Autodesk Fusion 360 part; units mm, degrees
(part 3 of 8)
  spline S66 degree 5 poles (224.4196, 240.1258) (224.453, 240.0356) (224.5199, 239.8554) (224.6207, 239.5853) (224.756, 239.2258) (224.9266, 238.7773) (225.0987, 238.3298) (225.2723, 237.8833) (225.4474, 237.4376) (225.624, 236.993) (225.802, 236.5493) (225.9816, 236.1066) (226.1627, 235.665) (226.3454, 235.2243) (226.5295, 234.7846) (226.7152, 234.346) (226.9025, 233.9085) (227.0914, 233.472) (227.2818, 233.0365) (227.4737, 232.6022) (227.6673, 232.1689) (227.8625, 231.7368) (228.0592, 231.3057) (228.2576, 230.8758) (228.4577, 230.4471) (228.6593, 230.0195) (228.8626, 229.5931) (229.0676, 229.1679) (229.2743, 228.7439) (229.4826, 228.3212) (229.6927, 227.8997) (229.9044, 227.4794) (230.1179, 227.0605) (230.3331, 226.6428) (230.5501, 226.2264) (230.7689, 225.8114) (230.9894, 225.3978) (231.2118, 224.9856) (231.436, 224.5747) (231.6621, 224.1653) (231.89, 223.7574) (232.1198, 223.3509) (232.3515, 222.9459) (232.5851, 222.5425) (232.8207, 222.1406) (233.0583, 221.7403) (233.2979, 221.3417) (233.5396, 220.9447) (233.7833, 220.5495) (234.0292, 220.1561) (234.2772, 219.7644) (234.5273, 219.3745) (234.7796, 218.9864) (235.0342, 218.6002) (235.2911, 218.216) (235.5503, 217.8339) (235.8121, 217.454) (236.0764, 217.0763) (236.3433, 216.701) (236.6129, 216.3281) (236.8851, 215.9574) (237.1217, 215.6404) (237.3048, 215.3984) (237.4332, 215.2303) (237.5062, 215.1354) (237.5232, 215.1133) knots -1 -1 -1 -1 -1 -1 -0.98571429 -0.97142857 -0.95714286 -0.94285714 -0.92857143 -0.91428571 -0.9 -0.88571429 -0.87142857 -0.85714286 -0.84285714 -0.82857143 -0.81428571 -0.8 -0.78571429 -0.77142857 -0.75714286 -0.74285714 -0.72857143 -0.71428571 -0.7 -0.68571429 -0.67142857 -0.65714286 -0.64285714 -0.62857143 -0.61428571 -0.6 -0.58571429 -0.57142857 -0.55714286 -0.54285714 -0.52857143 -0.51428571 -0.5 -0.48571429 -0.47142857 -0.45714286 -0.44285714 -0.42857143 -0.41428571 -0.4 -0.38571429 -0.37142857 -0.35714286 -0.34285714 -0.32857143 -0.31428571 -0.3 -0.28571429 -0.27142857 -0.25714286 -0.24285714 -0.22857143 -0.21428571 -0.2 -0.18571429 -0.17142857 -0.15714286 -0.14285714 -0.13851185 -0.13851185 -0.13851185 -0.13851185 -0.13851185 -0.13851185
  spline S67 degree 3 poles (237.4436, 213.0816) (237.5821, 213.235) (237.6893, 213.4141) (237.829, 213.8032) (237.8602, 214.0095) (237.8437, 214.3779) (237.8118, 214.5377) (237.7006, 214.8421) (237.622, 214.9849) (237.5232, 215.1133) knots 0 0 0 0 0.062015 0.062015 0.12403 0.12403 0.172638 0.172638 0.221247 0.221247 0.221247 0.221247
  arc A34 (237.4436, 213.0816) -> (232.0105, 206.8863) centre (452.3696, 19.1166) ccw
  spline S68 degree 3 poles (230.0066, 206.5422) (230.1854, 206.4386) (230.3829, 206.3709) (230.7925, 206.3151) (231.0008, 206.3274) (231.3577, 206.42) (231.5074, 206.4845) (231.7821, 206.6565) (231.9054, 206.763) (232.0105, 206.8863) knots 0 0 0 0 0.062015 0.062015 0.12403 0.12403 0.172638 0.172638 0.221247 0.221247 0.221247 0.221247
  spline S69 degree 5 poles (230.0066, 206.5422) (229.9824, 206.5562) (229.8788, 206.6161) (229.6954, 206.7215) (229.4315, 206.8714) (229.0863, 207.0646) (228.6834, 207.2861) (228.2784, 207.5047) (227.8715, 207.7204) (227.4625, 207.9332) (227.0517, 208.1431) (226.639, 208.3503) (226.2246, 208.5548) (225.8085, 208.7567) (225.3908, 208.9563) (224.9716, 209.1534) (224.5509, 209.3481) (224.1287, 209.5405) (223.705, 209.7306) (223.2799, 209.9184) (222.8534, 210.1039) (222.4256, 210.2872) (221.9964, 210.4683) (221.5659, 210.6473) (221.1341, 210.8242) (220.7012, 210.9989) (220.2669, 211.1717) (219.8315, 211.3423) (219.3949, 211.511) (218.9572, 211.6777) (218.5183, 211.8423) (218.0783, 212.0051) (217.6372, 212.1659) (217.195, 212.3247) (216.7518, 212.4817) (216.3075, 212.6368) (215.8621, 212.79) (215.4158, 212.9414) (214.9685, 213.0909) (214.5202, 213.2387) (214.0709, 213.3846) (213.6206, 213.5287) (213.1695, 213.6711) (212.7173, 213.8116) (212.2643, 213.9505) (211.8104, 214.0876) (211.3556, 214.2229) (210.8999, 214.3566) (210.4433, 214.4885) (209.9859, 214.6188) (209.5276, 214.7473) (209.0685, 214.8742) (208.6086, 214.9994) (208.1479, 215.123) (207.6863, 215.2449) (207.224, 215.3651) (206.7609, 215.4838) (206.297, 215.6008) (205.8323, 215.7162) (205.3669, 215.83) (204.9008, 215.9422) (204.4339, 216.0528) (204.0598, 216.1401) (203.7789, 216.2048) (203.5914, 216.2476) (203.4977, 216.2689) knots 0.13851185 0.13851185 0.13851185 0.13851185 0.13851185 0.13851185 0.14285714 0.15714286 0.17142857 0.18571429 0.2 0.21428571 0.22857143 0.24285714 0.25714286 0.27142857 0.28571429 0.3 0.31428571 0.32857143 0.34285714 0.35714286 0.37142857 0.38571429 0.4 0.41428571 0.42857143 0.44285714 0.45714286 0.47142857 0.48571429 0.5 0.51428571 0.52857143 0.54285714 0.55714286 0.57142857 0.58571429 0.6 0.61428571 0.62857143 0.64285714 0.65714286 0.67142857 0.68571429 0.7 0.71428571 0.72857143 0.74285714 0.75714286 0.77142857 0.78571429 0.8 0.81428571 0.82857143 0.84285714 0.85714286 0.87142857 0.88571429 0.9 0.91428571 0.92857143 0.94285714 0.95714286 0.97142857 0.98571429 1 1 1 1 1 1
  arc A35 (203.4977, 216.2689) -> (197.5222, 208.4816) centre (452.3696, 19.1166) ccw
  spline S70 degree 5 poles (197.5222, 208.4816) (197.5671, 208.3965) (197.657, 208.2266) (197.7922, 207.972) (197.9733, 207.6332) (198.201, 207.2109) (198.43, 206.7896) (198.6604, 206.3695) (198.8921, 205.9506) (199.1252, 205.5328) (199.3597, 205.1162) (199.5955, 204.7007) (199.8327, 204.2864) (200.0713, 203.8734) (200.3113, 203.4615) (200.5527, 203.0509) (200.7955, 202.6415) (201.0396, 202.2334) (201.2853, 201.8266) (201.5323, 201.421) (201.7808, 201.0167) (202.0307, 200.6137) (202.282, 200.2121) (202.5348, 199.8117) (202.7891, 199.4128) (203.0448, 199.0152) (203.3021, 198.619) (203.5608, 198.2242) (203.821, 197.8308) (204.0828, 197.4388) (204.346, 197.0483) (204.6108, 196.6593) (204.8772, 196.2718) (205.1451, 195.8858) (205.4145, 195.5013) (205.6856, 195.1184) (205.9583, 194.7371) (206.2326, 194.3574) (206.5085, 193.9794) (206.786, 193.603) (207.0652, 193.2283) (207.3461, 192.8553) (207.6287, 192.484) (207.913, 192.1145) (208.199, 191.7468) (208.4868, 191.381) (208.7764, 191.017) (209.0678, 190.655) (209.3611, 190.295) (209.6562, 189.937) (209.9532, 189.581) (210.2521, 189.2271) (210.5529, 188.8753) (210.8557, 188.5257) (211.1605, 188.1783) (211.4674, 187.8333) (211.7765, 187.4907) (212.0879, 187.1508) (212.4015, 186.8136) (212.7175, 186.479) (213.0357, 186.1471) (213.3117, 185.8637) (213.5248, 185.6476) (213.6741, 185.4977) (213.7588, 185.4131) (213.7785, 185.3934) knots -1 -1 -1 -1 -1 -1 -0.98571429 -0.97142857 -0.95714286 -0.94285714 -0.92857143 -0.91428571 -0.9 -0.88571429 -0.87142857 -0.85714286 -0.84285714 -0.82857143 -0.81428571 -0.8 -0.78571429 -0.77142857 -0.75714286 -0.74285714 -0.72857143 -0.71428571 -0.7 -0.68571429 -0.67142857 -0.65714286 -0.64285714 -0.62857143 -0.61428571 -0.6 -0.58571429 -0.57142857 -0.55714286 -0.54285714 -0.52857143 -0.51428571 -0.5 -0.48571429 -0.47142857 -0.45714286 -0.44285714 -0.42857143 -0.41428571 -0.4 -0.38571429 -0.37142857 -0.35714286 -0.34285714 -0.32857143 -0.31428571 -0.3 -0.28571429 -0.27142857 -0.25714286 -0.24285714 -0.22857143 -0.21428571 -0.2 -0.18571429 -0.17142857 -0.15714286 -0.14285714 -0.13851185 -0.13851185 -0.13851185 -0.13851185 -0.13851185 -0.13851185
  spline S71 degree 3 poles (213.9648, 183.3687) (214.0821, 183.5389) (214.165, 183.7304) (214.2527, 184.1344) (214.2567, 184.3431) (214.1923, 184.7062) (214.1398, 184.8604) (213.9898, 185.1477) (213.8933, 185.279) (213.7785, 185.3934) knots 0 0 0 0 0.062015 0.062015 0.12403 0.12403 0.172638 0.172638 0.221247 0.221247 0.221247 0.221247
  arc A36 (213.9648, 183.3687) -> (209.3868, 176.5173) centre (452.3696, 19.1166) ccw
  spline S72 degree 3 poles (207.445, 175.9146) (207.6358, 175.8352) (207.8404, 175.7939) (208.2538, 175.7919) (208.4587, 175.8314) (208.8005, 175.9698) (208.9405, 176.0532) (209.1904, 176.2596) (209.2988, 176.3813) (209.3868, 176.5173) knots 0 0 0 0 0.062015 0.062015 0.12403 0.12403 0.172638 0.172638 0.221247 0.221247 0.221247 0.221247
  spline S73 degree 5 poles (207.445, 175.9146) (207.4192, 175.9253) (207.3086, 175.9712) (207.113, 176.0517) (206.8318, 176.1659) (206.4644, 176.3124) (206.036, 176.4794) (205.606, 176.6433) (205.1743, 176.804) (204.7411, 176.9616) (204.3064, 177.1161) (203.8702, 177.2676) (203.4326, 177.4163) (202.9937, 177.5622) (202.5536, 177.7055) (202.1122, 177.8462) (201.6697, 177.9843) (201.226, 178.12) (200.7812, 178.2532) (200.3352, 178.3839) (199.8881, 178.5121) (199.44, 178.638) (198.9909, 178.7616) (198.5407, 178.8828) (198.0895, 179.0018) (197.6374, 179.1186) (197.1844, 179.2331) (196.7304, 179.3455) (196.2756, 179.4558) (195.8198, 179.5638) (195.3632, 179.6698) (194.9057, 179.7737) (194.4474, 179.8756) (193.9882, 179.9754) (193.5283, 180.0731) (193.0676, 180.1689) (192.606, 180.2627) (192.1438, 180.3545) (191.6807, 180.4444) (191.217, 180.5324) (190.7525, 180.6184) (190.2873, 180.7025) (189.8214, 180.7847) (189.3548, 180.8651) (188.8875, 180.9436) (188.4196, 181.0203) (187.951, 181.0951) (187.4818, 181.1681) (187.0119, 181.2394) (186.5414, 181.3088) (186.0702, 181.3764) (185.5985, 181.4423) (185.1262, 181.5064) (184.6533, 181.5688) (184.1797, 181.6294) (183.7057, 181.6883) (183.231, 181.7454) (182.7558, 181.8009) (182.2801, 181.8547) (181.8038, 181.9068) (181.327, 181.9572) (180.8497, 182.0059) (180.4674, 182.0436) (180.1804, 182.0711) (179.989, 182.089) (179.8933, 182.098) knots 0.13851185 0.13851185 0.13851185 0.13851185 0.13851185 0.13851185 0.14285714 0.15714286 0.17142857 0.18571429 0.2 0.21428571 0.22857143 0.24285714 0.25714286 0.27142857 0.28571429 0.3 0.31428571 0.32857143 0.34285714 0.35714286 0.37142857 0.38571429 0.4 0.41428571 0.42857143 0.44285714 0.45714286 0.47142857 0.48571429 0.5 0.51428571 0.52857143 0.54285714 0.55714286 0.57142857 0.58571429 0.6 0.61428571 0.62857143 0.64285714 0.65714286 0.67142857 0.68571429 0.7 0.71428571 0.72857143 0.74285714 0.75714286 0.77142857 0.78571429 0.8 0.81428571 0.82857143 0.84285714 0.85714286 0.87142857 0.88571429 0.9 0.91428571 0.92857143 0.94285714 0.95714286 0.97142857 0.98571429 1 1 1 1 1 1
  arc A37 (179.8933, 182.098) -> (174.9854, 173.5973) centre (452.3696, 19.1166) ccw
  spline S74 degree 5 poles (174.9854, 173.5973) (175.041, 173.5188) (175.1523, 173.3621) (175.3196, 173.1273) (175.5433, 172.8151) (175.8242, 172.426) (176.1062, 172.0383) (176.3895, 171.6519) (176.6739, 171.2668) (176.9596, 170.883) (177.2464, 170.5005) (177.5344, 170.1194) (177.8237, 169.7396) (178.1142, 169.3612) (178.4058, 168.9842) (178.6988, 168.6086) (178.9929, 168.2344) (179.2883, 167.8617) (179.5849, 167.4904) (179.8827, 167.1205) (180.1819, 166.7521) (180.4822, 166.3852) (180.7838, 166.0198) (181.0867, 165.6559) (181.3909, 165.2935) (181.6964, 164.9327) (182.0031, 164.5735) (182.3112, 164.2158) (182.6205, 163.8598) (182.9312, 163.5053) (183.2431, 163.1525) (183.5565, 162.8014) (183.8711, 162.452) (184.1871, 162.1043) (184.5045, 161.7583) (184.8232, 161.414) (185.1433, 161.0716) (185.4648, 160.7309) (185.7877, 160.3921) (186.112, 160.0551) (186.4377, 159.7201) (186.7649, 159.3869) (187.0935, 159.0557) (187.4236, 158.7265) (187.7552, 158.3993) (188.0883, 158.0741) (188.4229, 157.7511) (188.759, 157.4302) (189.0968, 157.1116) (189.4361, 156.7952) (189.777, 156.481) (190.1196, 156.1691) (190.4637, 155.8596) (190.8096, 155.5525) (191.1571, 155.2478) (191.5064, 154.9458) (191.8576, 154.6466) (192.2106, 154.3502) (192.5656, 154.0568) (192.9226, 153.7663) (193.2814, 153.4788) (193.592, 153.2338) (193.8315, 153.0474) (193.999, 152.9183) (194.0941, 152.8455) (194.1162, 152.8285) knots -1 -1 -1 -1 -1 -1 -0.98571429 -0.97142857 -0.95714286 -0.94285714 -0.92857143 -0.91428571 -0.9 -0.88571429 -0.87142857 -0.85714286 -0.84285714 -0.82857143 -0.81428571 -0.8 -0.78571429 -0.77142857 -0.75714286 -0.74285714 -0.72857143 -0.71428571 -0.7 -0.68571429 -0.67142857 -0.65714286 -0.64285714 -0.62857143 -0.61428571 -0.6 -0.58571429 -0.57142857 -0.55714286 -0.54285714 -0.52857143 -0.51428571 -0.5 -0.48571429 -0.47142857 -0.45714286 -0.44285714 -0.42857143 -0.41428571 -0.4 -0.38571429 -0.37142857 -0.35714286 -0.34285714 -0.32857143 -0.31428571 -0.3 -0.28571429 -0.27142857 -0.25714286 -0.24285714 -0.22857143 -0.21428571 -0.2 -0.18571429 -0.17142857 -0.15714286 -0.14285714 -0.13851185 -0.13851185 -0.13851185 -0.13851185 -0.13851185 -0.13851185
  spline S75 degree 3 poles (194.5652, 150.8454) (194.6592, 151.0295) (194.7165, 151.2302) (194.7507, 151.6422) (194.7274, 151.8496) (194.6162, 152.2012) (194.544, 152.3472) (194.3578, 152.6125) (194.2449, 152.7301) (194.1162, 152.8285) knots 0 0 0 0 0.062015 0.062015 0.12403 0.12403 0.172638 0.172638 0.221247 0.221247 0.221247 0.221247
  arc A38 (194.5652, 150.8454) -> (190.9207, 143.4551) centre (452.3696, 19.1166) ccw
  spline S76 degree 3 poles (189.0741, 142.6041) (189.2737, 142.5503) (189.4819, 142.536) (189.892, 142.5881) (190.09, 142.6539) (190.4108, 142.8357) (190.5387, 142.9367) (190.7595, 143.174) (190.8511, 143.3088) (190.9207, 143.4551) knots 0 0 0 0 0.062015 0.062015 0.12403 0.12403 0.172638 0.172638 0.221247 0.221247 0.221247 0.221247
  spline S77 degree 5 poles (189.0741, 142.6041) (189.0471, 142.6113) (188.9315, 142.6424) (188.7271, 142.6967) (188.4334, 142.7732) (188.05, 142.8705) (187.6034, 142.9802) (187.1557, 143.0865) (186.7068, 143.1895) (186.2567, 143.2892) (185.8056, 143.3856) (185.3533, 143.4789) (184.9001, 143.5692) (184.4459, 143.6566) (183.9908, 143.7412) (183.5348, 143.8231) (183.0781, 143.9023) (182.6205, 143.9789) (182.162, 144.0528) (181.7028, 144.1242) (181.2429, 144.193) (180.7821, 144.2593) (180.3207, 144.3232) (179.8586, 144.3847) (179.3957, 144.4438) (178.9323, 144.5005) (178.4681, 144.555) (178.0034, 144.6071) (177.538, 144.6571) (177.0721, 144.7047) (176.6055, 144.7502) (176.1384, 144.7935) (175.6707, 144.8347) (175.2024, 144.8737) (174.7337, 144.9106) (174.2644, 144.9454) (173.7946, 144.9781) (173.3243, 145.0088) (172.8535, 145.0375) (172.3822, 145.0642) (171.9105, 145.0888) (171.4383, 145.1115) (170.9656, 145.1322) (170.4925, 145.151) (170.019, 145.1679) (169.545, 145.1828) (169.0707, 145.1958) (168.5959, 145.207) (168.1208, 145.2163) (167.6452, 145.2237) (167.1693, 145.2292) (166.693, 145.233) (166.2164, 145.2349) (165.7393, 145.235) (165.262, 145.2333) (164.7843, 145.2298) (164.3062, 145.2245) (163.8278, 145.2175) (163.3491, 145.2087) (162.8701, 145.1982) (162.3908, 145.1859) (161.9112, 145.1719) (161.5273, 145.1593) (161.2392, 145.1491) (161.0471, 145.142) (160.951, 145.1383) knots 0.13851185 0.13851185 0.13851185 0.13851185 0.13851185 0.13851185 0.14285714 0.15714286 0.17142857 0.18571429 0.2 0.21428571 0.22857143 0.24285714 0.25714286 0.27142857 0.28571429 0.3 0.31428571 0.32857143 0.34285714 0.35714286 0.37142857 0.38571429 0.4 0.41428571 0.42857143 0.44285714 0.45714286 0.47142857 0.48571429 0.5 0.51428571 0.52857143 0.54285714 0.55714286 0.57142857 0.58571429 0.6 0.61428571 0.62857143 0.64285714 0.65714286 0.67142857 0.68571429 0.7 0.71428571 0.72857143 0.74285714 0.75714286 0.77142857 0.78571429 0.8 0.81428571 0.82857143 0.84285714 0.85714286 0.87142857 0.88571429 0.9 0.91428571 0.92857143 0.94285714 0.95714286 0.97142857 0.98571429 1 1 1 1 1 1
  arc A39 (160.951, 145.1383) -> (157.1947, 136.0698) centre (452.3696, 19.1166) ccw
  spline S78 degree 5 poles (157.1947, 136.0698) (157.26, 135.9993) (157.3908, 135.8584) (157.5873, 135.6474) (157.8499, 135.3671) (158.1792, 135.018) (158.5094, 134.6704) (158.8407, 134.3243) (159.173, 133.9796) (159.5062, 133.6364) (159.8405, 133.2946) (160.1759, 132.9543) (160.5122, 132.6156) (160.8496, 132.2784) (161.188, 131.9427) (161.5274, 131.6085) (161.8679, 131.2759) (162.2094, 130.9449) (162.5519, 130.6155) (162.8955, 130.2876) (163.2402, 129.9614) (163.5858, 129.6369) (163.9326, 129.314) (164.2804, 128.9927) (164.6293, 128.6731) (164.9792, 128.3553) (165.3302, 128.0392) (165.6823, 127.7248) (166.0355, 127.4121) (166.3897, 127.1013) (166.7451, 126.7922) (167.1016, 126.485) (167.4591, 126.1796) (167.8178, 125.8761) (168.1776, 125.5745) (168.5385, 125.2748) (168.9006, 124.9771) (169.2638, 124.6813) (169.6282, 124.3875) (169.9937, 124.0958) (170.3604, 123.8061) (170.7282, 123.5185) (171.0973, 123.2331) (171.4675, 122.9497) (171.839, 122.6686) (172.2116, 122.3897) (172.5855, 122.1131) (172.9607, 121.8389) (173.3372, 121.567) (173.7149, 121.2976) (174.0939, 121.0306) (174.4742, 120.7661) (174.8558, 120.5042) (175.2388, 120.2448) (175.6231, 119.9881) (176.0089, 119.7343) (176.3961, 119.4835) (176.7848, 119.2357) (177.1751, 118.9911) (177.5668, 118.7497) (177.9602, 118.5115) (178.3001, 118.3092) (178.5618, 118.1556) (178.7448, 118.0495) (178.8485, 117.9897) (178.8727, 117.9758) knots -1 -1 -1 -1 -1 -1 -0.98571429 -0.97142857 -0.95714286 -0.94285714 -0.92857143 -0.91428571 -0.9 -0.88571429 -0.87142857 -0.85714286 -0.84285714 -0.82857143 -0.81428571 -0.8 -0.78571429 -0.77142857 -0.75714286 -0.74285714 -0.72857143 -0.71428571 -0.7 -0.68571429 -0.67142857 -0.65714286 -0.64285714 -0.62857143 -0.61428571 -0.6 -0.58571429 -0.57142857 -0.55714286 -0.54285714 -0.52857143 -0.51428571 -0.5 -0.48571429 -0.47142857 -0.45714286 -0.44285714 -0.42857143 -0.41428571 -0.4 -0.38571429 -0.37142857 -0.35714286 -0.34285714 -0.32857143 -0.31428571 -0.3 -0.28571429 -0.27142857 -0.25714286 -0.24285714 -0.22857143 -0.21428571 -0.2 -0.18571429 -0.17142857 -0.15714286 -0.14285714 -0.13851185 -0.13851185 -0.13851185 -0.13851185 -0.13851185 -0.13851185
  spline S79 degree 3 poles (179.5767, 116.0682) (179.6459, 116.263) (179.6764, 116.4695) (179.6566, 116.8824) (179.6065, 117.085) (179.4503, 117.419) (179.3596, 117.5544) (179.1404, 117.7931) (179.0131, 117.8949) (178.8727, 117.9758) knots 0 0 0 0 0.062015 0.062015 0.12403 0.12403 0.172638 0.172638 0.221247 0.221247 0.221247 0.221247
  arc A40 (179.5767, 116.0682) -> (176.928, 108.2654) centre (452.3696, 19.1166) ccw
  spline S80 degree 3 poles (175.2083, 107.1806) (175.4132, 107.1534) (175.6215, 107.1664) (176.0213, 107.2716) (176.209, 107.3627) (176.5033, 107.5848) (176.617, 107.7017) (176.8049, 107.9657) (176.8781, 108.1113) (176.928, 108.2654) knots 0 0 0 0 0.062015 0.062015 0.12403 0.12403 0.172638 0.172638 0.221247 0.221247 0.221247 0.221247
  spline S81 degree 5 poles (175.2083, 107.1806) (175.1806, 107.1843) (175.0619, 107.2) (174.8521, 107.2272) (174.551, 107.2648) (174.1582, 107.3112) (173.7011, 107.3616) (173.2433, 107.4086) (172.7848, 107.4521) (172.3256, 107.4922) (171.8657, 107.5289) (171.4051, 107.5624) (170.944, 107.5927) (170.4823, 107.6201) (170.02, 107.6446) (169.5573, 107.6662) (169.0941, 107.6852) (168.6304, 107.7013) (168.1662, 107.7148) (167.7017, 107.7257) (167.2366, 107.7338) (166.7712, 107.7395) (166.3054, 107.7426) (165.8392, 107.7432) (165.3726, 107.7413) (164.9057, 107.7371) (164.4384, 107.7305) (163.9708, 107.7216) (163.5029, 107.7103) (163.0347, 107.6968) (162.5662, 107.681) (162.0974, 107.6629) (161.6284, 107.6427) (161.1591, 107.6202) (160.6895, 107.5956) (160.2196, 107.5689) (159.7496, 107.54) (159.2793, 107.5091) (158.8088, 107.4761) (158.3381, 107.441) (157.8671, 107.4039) (157.396, 107.3647) (156.9247, 107.3236) (156.4532, 107.2804) (155.9815, 107.2353) (155.5097, 107.1883) (155.0377, 107.1393) (154.5656, 107.0884) (154.0933, 107.0355) (153.6208, 106.9808) (153.1482, 106.9242) (152.6755, 106.8658) (152.2027, 106.8054) (151.7297, 106.7433) (151.2567, 106.6793) (150.7835, 106.6134) (150.3102, 106.5458) (149.8369, 106.4764) (149.3634, 106.4052) (148.8899, 106.3323) (148.4163, 106.2575) (147.9426, 106.1811) (147.5636, 106.1185) (147.2793, 106.0708) (147.0898, 106.0386) (146.995, 106.0224) knots 0.13851185 0.13851185 0.13851185 0.13851185 0.13851185 0.13851185 0.14285714 0.15714286 0.17142857 0.18571429 0.2 0.21428571 0.22857143 0.24285714 0.25714286 0.27142857 0.28571429 0.3 0.31428571 0.32857143 0.34285714 0.35714286 0.37142857 0.38571429 0.4 0.41428571 0.42857143 0.44285714 0.45714286 0.47142857 0.48571429 0.5 0.51428571 0.52857143 0.54285714 0.55714286 0.57142857 0.58571429 0.6 0.61428571 0.62857143 0.64285714 0.65714286 0.67142857 0.68571429 0.7 0.71428571 0.72857143 0.74285714 0.75714286 0.77142857 0.78571429 0.8 0.81428571 0.82857143 0.84285714 0.85714286 0.87142857 0.88571429 0.9 0.91428571 0.92857143 0.94285714 0.95714286 0.97142857 0.98571429 1 1 1 1 1 1
  arc A41 (146.995, 106.0224) -> (144.4545, 96.5412) centre (452.3696, 19.1166) ccw
  spline S82 degree 5 poles (144.4545, 96.5412) (144.5285, 96.4798) (144.6766, 96.3572) (144.8989, 96.1737) (145.1958, 95.93) (145.5678, 95.6269) (145.9406, 95.3254) (146.3142, 95.0255) (146.6887, 94.7271) (147.0639, 94.4303) (147.44, 94.1351) (147.8168, 93.8415) (148.1945, 93.5496) (148.573, 93.2592) (148.9523, 92.9706) (149.3325, 92.6836) (149.7134, 92.3983) (150.0952, 92.1147) (150.4778, 91.8328) (150.8613, 91.5526) (151.2455, 91.2742) (151.6306, 90.9975) (152.0166, 90.7226) (152.4033, 90.4495) (152.7909, 90.1782) (153.1793, 89.9088) (153.5686, 89.6412) (153.9587, 89.3754) (154.3497, 89.1116) (154.7415, 88.8496) (155.1342, 88.5896) (155.5277, 88.3315) (155.922, 88.0754) (156.3173, 87.8213) (156.7134, 87.5693) (157.1103, 87.3192) (157.5081, 87.0713) (157.9068, 86.8255) (158.3064, 86.5818) (158.7069, 86.3402) (159.1083, 86.1009) (159.5105, 85.8638) (159.9137, 85.6289) (160.3177, 85.3963) (160.7227, 85.1661) (161.1286, 84.9382) (161.5354, 84.7128) (161.9431, 84.4899) (162.3518, 84.2695) (162.7615, 84.0517) (163.1721, 83.8365) (163.5837, 83.6239) (163.9963, 83.414) (164.4098, 83.2068) (164.8243, 83.0025) (165.2399, 82.8012) (165.6566, 82.6031) (166.0743, 82.4082) (166.4931, 82.2166) (166.9131, 82.0284) (167.3341, 81.8436) (167.6975, 81.6873) (167.9771, 81.5693) (168.1724, 81.4879) (168.283, 81.4422) (168.3088, 81.4315) knots -1 -1 -1 -1 -1 -1 -0.98571429 -0.97142857 -0.95714286 -0.94285714 -0.92857143 -0.91428571 -0.9 -0.88571429 -0.87142857 -0.85714286 -0.84285714 -0.82857143 -0.81428571 -0.8 -0.78571429 -0.77142857 -0.75714286 -0.74285714 -0.72857143 -0.71428571 -0.7 -0.68571429 -0.67142857 -0.65714286 -0.64285714 -0.62857143 -0.61428571 -0.6 -0.58571429 -0.57142857 -0.55714286 -0.54285714 -0.52857143 -0.51428571 -0.5 -0.48571429 -0.47142857 -0.45714286 -0.44285714 -0.42857143 -0.41428571 -0.4 -0.38571429 -0.37142857 -0.35714286 -0.34285714 -0.32857143 -0.31428571 -0.3 -0.28571429 -0.27142857 -0.25714286 -0.24285714 -0.22857143 -0.21428571 -0.2 -0.18571429 -0.17142857 -0.15714286 -0.14285714 -0.13851185 -0.13851185 -0.13851185 -0.13851185 -0.13851185 -0.13851185
  spline S83 degree 3 poles (169.2557, 79.6322) (169.2989, 79.8343) (169.3022, 80.043) (169.2287, 80.4498) (169.1526, 80.6441) (168.9541, 80.9549) (168.8465, 81.0773) (168.598, 81.2853) (168.4586, 81.3697) (168.3088, 81.4315) knots 0 0 0 0 0.062015 0.062015 0.12403 0.12403 0.172638 0.172638 0.221247 0.221247 0.221247 0.221247
  arc A42 (169.2557, 79.6322) -> (167.6482, 71.5504) centre (452.3696, 19.1166) ccw
  spline S84 degree 3 poles (166.0848, 70.2504) (166.2915, 70.2502) (166.4963, 70.2903) (166.879, 70.4467) (167.0532, 70.5615) (167.316, 70.8202) (167.4134, 70.9509) (167.5652, 71.2372) (167.6188, 71.3911) (167.6482, 71.5504) knots 0 0 0 0 0.062015 0.062015 0.12403 0.12403 0.172638 0.172638 0.221247 0.221247 0.221247 0.221247
  spline S85 degree 5 poles (166.0848, 70.2504) (166.0568, 70.2505) (165.9371, 70.2506) (165.7256, 70.2501) (165.4221, 70.248) (165.0266, 70.2428) (164.5669, 70.2331) (164.1069, 70.2199) (163.6466, 70.2032) (163.1861, 70.183) (162.7253, 70.1594) (162.2643, 70.1325) (161.8032, 70.1024) (161.3418, 70.0692) (160.8803, 70.0332) (160.4187, 69.9943) (159.957, 69.9526) (159.4952, 69.9081) (159.0333, 69.8609) (158.5712, 69.811) (158.1091, 69.7584) (157.6469, 69.7032) (157.1847, 69.6455) (156.7224, 69.5852) (156.26, 69.5225) (155.7977, 69.4574) (155.3353, 69.3899) (154.8728, 69.32) (154.4104, 69.2477) (153.948, 69.1732) (153.4856, 69.0964) (153.0231, 69.0173) (152.5607, 68.936) (152.0984, 68.8525) (151.636, 68.7668) (151.1737, 68.679) (150.7114, 68.589) (150.2492, 68.4969) (149.787, 68.4028) (149.3249, 68.3065) (148.8629, 68.2083) (148.4009, 68.108) (147.939, 68.0057) (147.4771, 67.9014) (147.0154, 67.7951) (146.5537, 67.6868) (146.0922, 67.5766) (145.6307, 67.4645) (145.1693, 67.3505) (144.7081, 67.2346) (144.2469, 67.1168) (143.7859, 66.9971) (143.325, 66.8756) (142.8642, 66.7522) (142.4035, 66.627) (141.943, 66.5) (141.4826, 66.3712) (141.0223, 66.2406) (140.5622, 66.1082) (140.1023, 65.9741) (139.6425, 65.8382) (139.1828, 65.7005) (138.8152, 65.589) (138.5396, 65.5046) (138.3559, 65.448) (138.264, 65.4196) knots 0.13851185 0.13851185 0.13851185 0.13851185 0.13851185 0.13851185 0.14285714 0.15714286 0.17142857 0.18571429 0.2 0.21428571 0.22857143 0.24285714 0.25714286 0.27142857 0.28571429 0.3 0.31428571 0.32857143 0.34285714 0.35714286 0.37142857 0.38571429 0.4 0.41428571 0.42857143 0.44285714 0.45714286 0.47142857 0.48571429 0.5 0.51428571 0.52857143 0.54285714 0.55714286 0.57142857 0.58571429 0.6 0.61428571 0.62857143 0.64285714 0.65714286 0.67142857 0.68571429 0.7 0.71428571 0.72857143 0.74285714 0.75714286 0.77142857 0.78571429 0.8 0.81428571 0.82857143 0.84285714 0.85714286 0.87142857 0.88571429 0.9 0.91428571 0.92857143 0.94285714 0.95714286 0.97142857 0.98571429 1 1 1 1 1 1
  arc A43 (138.264, 65.4196) -> (136.9828, 55.6878) centre (452.3696, 19.1166) ccw
  spline S86 degree 5 poles (136.9828, 55.6878) (137.0642, 55.6366) (137.227, 55.5344) (137.4714, 55.3815) (137.7976, 55.1786) (138.206, 54.9267) (138.6149, 54.6764) (139.0245, 54.4278) (139.4347, 54.1809) (139.8454, 53.9356) (140.2568, 53.692) (140.6687, 53.4501) (141.0813, 53.21) (141.4945, 52.9715) (141.9082, 52.7349) (142.3226, 52.4999) (142.7375, 52.2668) (143.1531, 52.0355) (143.5692, 51.8059) (143.9859, 51.5782) (144.4032, 51.3523) (144.8212, 51.1283) (145.2397, 50.9061) (145.6588, 50.6858) (146.0784, 50.4674) (146.4987, 50.251) (146.9196, 50.0365) (147.3411, 49.8239) (147.7631, 49.6133) (148.1858, 49.4048) (148.609, 49.1982) (149.0328, 48.9937) (149.4573, 48.7913) (149.8823, 48.591) (150.3079, 48.3928) (150.7341, 48.1967) (151.1609, 48.0028) (151.5882, 47.8111) (152.0162, 47.6217) (152.4448, 47.4345) (152.8739, 47.2496) (153.3037, 47.067) (153.7341, 46.8867) (154.165, 46.7089) (154.5966, 46.5335) (155.0287, 46.3606) (155.4615, 46.1902) (155.8949, 46.0224) (156.3288, 45.8572) (156.7634, 45.6947) (157.1986, 45.5349) (157.6344, 45.3779) (158.0708, 45.2236) (158.5079, 45.0722) (158.9455, 44.9238) (159.3838, 44.7784) (159.8228, 44.6364) (160.2624, 44.4977) (160.7026, 44.3624) (161.1436, 44.2306) (161.5851, 44.1023) (161.9658, 43.9949) (162.2584, 43.9143) (162.4626, 43.8591) (162.5783, 43.8282) (162.6053, 43.821) knots -1 -1 -1 -1 -1 -1 -0.98571429 -0.97142857 -0.95714286 -0.94285714 -0.92857143 -0.91428571 -0.9 -0.88571429 -0.87142857 -0.85714286 -0.84285714 -0.82857143 -0.81428571 -0.8 -0.78571429 -0.77142857 -0.75714286 -0.74285714 -0.72857143 -0.71428571 -0.7 -0.68571429 -0.67142857 -0.65714286 -0.64285714 -0.62857143 -0.61428571 -0.6 -0.58571429 -0.57142857 -0.55714286 -0.54285714 -0.52857143 -0.51428571 -0.5 -0.48571429 -0.47142857 -0.45714286 -0.44285714 -0.42857143 -0.41428571 -0.4 -0.38571429 -0.37142857 -0.35714286 -0.34285714 -0.32857143 -0.31428571 -0.3 -0.28571429 -0.27142857 -0.25714286 -0.24285714 -0.22857143 -0.21428571 -0.2 -0.18571429 -0.17142857 -0.15714286 -0.14285714 -0.13851185 -0.13851185 -0.13851185 -0.13851185 -0.13851185 -0.13851185
  spline S87 degree 3 poles (163.7789, 42.1607) (163.7954, 42.3668) (163.7714, 42.5741) (163.6454, 42.9678) (163.5446, 43.1505) (163.3072, 43.4328) (163.1846, 43.5401) (162.9111, 43.7139) (162.7618, 43.7793) (162.6053, 43.821) knots 0 0 0 0 0.062015 0.062015 0.12403 0.12403 0.172638 0.172638 0.221247 0.221247 0.221247 0.221247
  arc A44 (163.7789, 42.1607) -> (163.24, 33.9382) centre (452.3696, 19.1166) ccw
  spline S88 degree 3 poles (161.8596, 32.4453) (162.0646, 32.472) (162.2624, 32.5385) (162.6214, 32.7436) (162.7792, 32.8802) (163.006, 33.1709) (163.0855, 33.3132) (163.1987, 33.6168) (163.2317, 33.7764) (163.24, 33.9382) knots 0 0 0 0 0.062015 0.062015 0.12403 0.12403 0.172638 0.172638 0.221247 0.221247 0.221247 0.221247
  spline S89 degree 5 poles (161.8596, 32.4453) (161.832, 32.4417) (161.7133, 32.4262) (161.5036, 32.3981) (161.203, 32.3564) (160.8115, 32.2996) (160.357, 32.23) (159.9027, 32.1569) (159.4485, 32.0803) (158.9946, 32.0001) (158.5408, 31.9166) (158.0873, 31.8297) (157.634, 31.7397) (157.181, 31.6466) (156.7281, 31.5506) (156.2756, 31.4518) (155.8232, 31.3502) (155.3711, 31.2458) (154.9193, 31.1387) (154.4678, 31.0289) (154.0165, 30.9165) (153.5654, 30.8014) (153.1147, 30.6838) (152.6642, 30.5638) (152.214, 30.4412) (151.7641, 30.3163) (151.3145, 30.189) (150.8651, 30.0594) (150.4161, 29.9274) (149.9673, 29.7931) (149.5189, 29.6566) (149.0707, 29.5178) (148.6229, 29.3769) (148.1754, 29.2337) (147.7282, 29.0884) (147.2813, 28.941) (146.8347, 28.7915) (146.3884, 28.6399) (145.9425, 28.4862) (145.4969, 28.3305) (145.0516, 28.1727) (144.6067, 28.013) (144.1621, 27.8512) (143.7178, 27.6875) (143.2739, 27.5219) (142.8303, 27.3543) (142.3871, 27.1848) (141.9442, 27.0135) (141.5017, 26.8402) (141.0595, 26.6651) (140.6177, 26.4881) (140.1762, 26.3093) (139.7351, 26.1286) (139.2943, 25.9461) (138.854, 25.7619) (138.414, 25.5759) (137.9743, 25.388) (137.535, 25.1985) (137.0962, 25.0072) (136.6576, 24.8142) (136.2195, 24.6194) (135.7818, 24.4229) (135.4319, 24.2644) (135.1696, 24.1447) (134.9948, 24.0646) (134.9075, 24.0244) knots 0.13851185 0.13851185 0.13851185 0.13851185 0.13851185 0.13851185 0.14285714 0.15714286 0.17142857 0.18571429 0.2 0.21428571 0.22857143 0.24285714 0.25714286 0.27142857 0.28571429 0.3 0.31428571 0.32857143 0.34285714 0.35714286 0.37142857 0.38571429 0.4 0.41428571 0.42857143 0.44285714 0.45714286 0.47142857 0.48571429 0.5 0.51428571 0.52857143 0.54285714 0.55714286 0.57142857 0.58571429 0.6 0.61428571 0.62857143 0.64285714 0.65714286 0.67142857 0.68571429 0.7 0.71428571 0.72857143 0.74285714 0.75714286 0.77142857 0.78571429 0.8 0.81428571 0.82857143 0.84285714 0.85714286 0.87142857 0.88571429 0.9 0.91428571 0.92857143 0.94285714 0.95714286 0.97142857 0.98571429 1 1 1 1 1 1
  arc A45 (134.9075, 24.0244) -> (134.9075, 14.2087) centre (452.3696, 19.1166) ccw
  spline S90 degree 5 poles (134.9075, 14.2087) (134.9948, 14.1686) (135.1696, 14.0885) (135.4319, 13.9688) (135.7818, 13.8102) (136.2195, 13.6138) (136.6576, 13.419) (137.0962, 13.226) (137.535, 13.0347) (137.9743, 12.8451) (138.414, 12.6573) (138.854, 12.4713) (139.2943, 12.287) (139.7351, 12.1046) (140.1762, 11.9239) (140.6177, 11.7451) (141.0595, 11.5681) (141.5017, 11.393) (141.9442, 11.2197) (142.3871, 11.0483) (142.8303, 10.8788) (143.2739, 10.7113) (143.7178, 10.5456) (144.1621, 10.3819) (144.6067, 10.2202) (145.0516, 10.0605) (145.4969, 9.9027) (145.9425, 9.747) (146.3884, 9.5933) (146.8347, 9.4417) (147.2813, 9.2922) (147.7282, 9.1448) (148.1754, 8.9995) (148.6229, 8.8563) (149.0707, 8.7153) (149.5189, 8.5766) (149.9673, 8.4401) (150.4161, 8.3058) (150.8651, 8.1738) (151.3145, 8.0442) (151.7641, 7.9169) (152.214, 7.7919) (152.6642, 7.6694) (153.1147, 7.5493) (153.5654, 7.4318) (154.0165, 7.3167) (154.4678, 7.2043) (154.9193, 7.0945) (155.3711, 6.9874) (155.8232, 6.883) (156.2756, 6.7814) (156.7281, 6.6826) (157.181, 6.5866) (157.634, 6.4935) (158.0873, 6.4035) (158.5408, 6.3166) (158.9946, 6.233) (159.4485, 6.1529) (159.9027, 6.0763) (160.357, 6.0032) (160.8115, 5.9336) (161.203, 5.8767) (161.5036, 5.8351) (161.7133, 5.807) (161.832, 5.7915) (161.8596, 5.7879) knots -1 -1 -1 -1 -1 -1 -0.98571429 -0.97142857 -0.95714286 -0.94285714 -0.92857143 -0.91428571 -0.9 -0.88571429 -0.87142857 -0.85714286 -0.84285714 -0.82857143 -0.81428571 -0.8 -0.78571429 -0.77142857 -0.75714286 -0.74285714 -0.72857143 -0.71428571 -0.7 -0.68571429 -0.67142857 -0.65714286 -0.64285714 -0.62857143 -0.61428571 -0.6 -0.58571429 -0.57142857 -0.55714286 -0.54285714 -0.52857143 -0.51428571 -0.5 -0.48571429 -0.47142857 -0.45714286 -0.44285714 -0.42857143 -0.41428571 -0.4 -0.38571429 -0.37142857 -0.35714286 -0.34285714 -0.32857143 -0.31428571 -0.3 -0.28571429 -0.27142857 -0.25714286 -0.24285714 -0.22857143 -0.21428571 -0.2 -0.18571429 -0.17142857 -0.15714286 -0.14285714 -0.13851185 -0.13851185 -0.13851185 -0.13851185 -0.13851185 -0.13851185
  spline S91 degree 3 poles (163.24, 4.2949) (163.2294, 4.5014) (163.1786, 4.7038) (163.0023, 5.0777) (162.8784, 5.2457) (162.6063, 5.4945) (162.4707, 5.5849) (162.1768, 5.7215) (162.0203, 5.7669) (161.8596, 5.7879) knots 0 0 0 0 0.062015 0.062015 0.12403 0.12403 0.172638 0.172638 0.221247 0.221247 0.221247 0.221247
  arc A46 (163.24, 4.2949) -> (163.7789, -3.9275) centre (452.3696, 19.1166) ccw
  spline S92 degree 3 poles (162.6053, -5.5879) (162.805, -5.5346) (162.9924, -5.4429) (163.3216, -5.1927) (163.4602, -5.0367) (163.6471, -4.7188) (163.7073, -4.5674) (163.7799, -4.2516) (163.7918, -4.089) (163.7789, -3.9275) knots 0 0 0 0 0.062015 0.062015 0.12403 0.12403 0.172638 0.172638 0.221247 0.221247 0.221247 0.221247
  spline S93 degree 5 poles (162.6053, -5.5879) (162.5783, -5.5951) (162.4626, -5.626) (162.2584, -5.6811) (161.9658, -5.7617) (161.5851, -5.8692) (161.1436, -5.9975) (160.7026, -6.1292) (160.2624, -6.2645) (159.8228, -6.4032) (159.3838, -6.5453) (158.9455, -6.6906) (158.5079, -6.839) (158.0708, -6.9904) (157.6344, -7.1447) (157.1986, -7.3018) (156.7634, -7.4616) (156.3288, -7.624) (155.8949, -7.7892) (155.4615, -7.957) (155.0287, -8.1274) (154.5966, -8.3003) (154.165, -8.4757) (153.7341, -8.6536) (153.3037, -8.8338) (152.8739, -9.0164) (152.4448, -9.2013) (152.0162, -9.3885) (151.5882, -9.5779) (151.1609, -9.7696) (150.7341, -9.9635) (150.3079, -10.1596) (149.8823, -10.3578) (149.4573, -10.5581) (149.0328, -10.7606) (148.609, -10.9651) (148.1858, -11.1716) (147.7631, -11.3802) (147.3411, -11.5907) (146.9196, -11.8033) (146.4987, -12.0178) (146.0784, -12.2343) (145.6588, -12.4526) (145.2397, -12.6729) (144.8212, -12.8951) (144.4032, -13.1191) (143.9859, -13.345) (143.5692, -13.5727) (143.1531, -13.8023) (142.7375, -14.0336) (142.3226, -14.2668) (141.9082, -14.5017) (141.4945, -14.7384) (141.0813, -14.9768) (140.6687, -15.217) (140.2568, -15.4588) (139.8454, -15.7024) (139.4347, -15.9477) (139.0245, -16.1946) (138.6149, -16.4433) (138.206, -16.6935) (137.7976, -16.9455) (137.4714, -17.1483) (137.227, -17.3012) (137.0642, -17.4034) (136.9828, -17.4547) knots 0.13851185 0.13851185 0.13851185 0.13851185 0.13851185 0.13851185 0.14285714 0.15714286 0.17142857 0.18571429 0.2 0.21428571 0.22857143 0.24285714 0.25714286 0.27142857 0.28571429 0.3 0.31428571 0.32857143 0.34285714 0.35714286 0.37142857 0.38571429 0.4 0.41428571 0.42857143 0.44285714 0.45714286 0.47142857 0.48571429 0.5 0.51428571 0.52857143 0.54285714 0.55714286 0.57142857 0.58571429 0.6 0.61428571 0.62857143 0.64285714 0.65714286 0.67142857 0.68571429 0.7 0.71428571 0.72857143 0.74285714 0.75714286 0.77142857 0.78571429 0.8 0.81428571 0.82857143 0.84285714 0.85714286 0.87142857 0.88571429 0.9 0.91428571 0.92857143 0.94285714 0.95714286 0.97142857 0.98571429 1 1 1 1 1 1
  arc A47 (136.9828, -17.4547) -> (138.264, -27.1864) centre (452.3696, 19.1166) ccw
  spline S94 degree 5 poles (138.264, -27.1864) (138.3559, -27.2148) (138.5396, -27.2714) (138.8152, -27.3558) (139.1828, -27.4674) (139.6425, -27.605) (140.1023, -27.7409) (140.5622, -27.8751) (141.0223, -28.0074) (141.4826, -28.138) (141.943, -28.2668) (142.4035, -28.3939) (142.8642, -28.5191) (143.325, -28.6424) (143.7859, -28.764) (144.2469, -28.8836) (144.7081, -29.0014) (145.1693, -29.1173) (145.6307, -29.2314) (146.0922, -29.3435) (146.5537, -29.4537) (147.0154, -29.5619) (147.4771, -29.6682) (147.939, -29.7725) (148.4009, -29.8748) (148.8629, -29.9751) (149.3249, -30.0734) (149.787, -30.1696) (150.2492, -30.2638) (150.7114, -30.3558) (151.1737, -30.4458) (151.636, -30.5336) (152.0984, -30.6193) (152.5607, -30.7028) (153.0231, -30.7841) (153.4856, -30.8632) (153.948, -30.94) (154.4104, -31.0146) (154.8728, -31.0868) (155.3353, -31.1567) (155.7977, -31.2242) (156.26, -31.2893) (156.7224, -31.3521) (157.1847, -31.4123) (157.6469, -31.47) (158.1091, -31.5252) (158.5712, -31.5778) (159.0333, -31.6277) (159.4952, -31.6749) (159.957, -31.7194) (160.4187, -31.7611) (160.8803, -31.8) (161.3418, -31.8361) (161.8032, -31.8692) (162.2643, -31.8993) (162.7253, -31.9262) (163.1861, -31.9499) (163.6466, -31.9701) (164.1069, -31.9868) (164.5669, -31.9999) (165.0266, -32.0096) (165.4221, -32.0149) (165.7256, -32.0169) (165.9371, -32.0174) (166.0568, -32.0173) (166.0848, -32.0173) knots -1 -1 -1 -1 -1 -1 -0.98571429 -0.97142857 -0.95714286 -0.94285714 -0.92857143 -0.91428571 -0.9 -0.88571429 -0.87142857 -0.85714286 -0.84285714 -0.82857143 -0.81428571 -0.8 -0.78571429 -0.77142857 -0.75714286 -0.74285714 -0.72857143 -0.71428571 -0.7 -0.68571429 -0.67142857 -0.65714286 -0.64285714 -0.62857143 -0.61428571 -0.6 -0.58571429 -0.57142857 -0.55714286 -0.54285714 -0.52857143 -0.51428571 -0.5 -0.48571429 -0.47142857 -0.45714286 -0.44285714 -0.42857143 -0.41428571 -0.4 -0.38571429 -0.37142857 -0.35714286 -0.34285714 -0.32857143 -0.31428571 -0.3 -0.28571429 -0.27142857 -0.25714286 -0.24285714 -0.22857143 -0.21428571 -0.2 -0.18571429 -0.17142857 -0.15714286 -0.14285714 -0.13851185 -0.13851185 -0.13851185 -0.13851185 -0.13851185 -0.13851185
  spline S95 degree 3 poles (167.6482, -33.3172) (167.6107, -33.114) (167.5339, -32.9199) (167.3103, -32.5722) (167.1656, -32.4218) (166.8633, -32.2106) (166.7171, -32.1387) (166.4079, -32.0416) (166.2468, -32.017) (166.0848, -32.0173) knots 0 0 0 0 0.062015 0.062015 0.12403 0.12403 0.172638 0.172638 0.221247 0.221247 0.221247 0.221247
  arc A48 (167.6482, -33.3172) -> (169.2557, -41.399) centre (452.3696, 19.1166) ccw
  spline S96 degree 3 poles (168.3088, -43.1983) (168.4999, -43.1195) (168.6738, -43.0041) (168.9674, -42.7131) (169.0845, -42.5403) (169.2283, -42.2008) (169.2683, -42.0428) (169.299, -41.7202) (169.2896, -41.5575) (169.2557, -41.399) knots 0 0 0 0 0.062015 0.062015 0.12403 0.12403 0.172638 0.172638 0.221247 0.221247 0.221247 0.221247
  spline S97 degree 5 poles (168.3088, -43.1983) (168.283, -43.209) (168.1724, -43.2547) (167.9771, -43.3361) (167.6975, -43.4541) (167.3341, -43.6104) (166.9131, -43.7952) (166.4931, -43.9834) (166.0743, -44.175) (165.6566, -44.3699) (165.2399, -44.568) (164.8243, -44.7693) (164.4098, -44.9736) (163.9963, -45.1808) (163.5837, -45.3907) (163.1721, -45.6033) (162.7615, -45.8185) (162.3518, -46.0363) (161.9431, -46.2567) (161.5354, -46.4797) (161.1286, -46.7051) (160.7227, -46.9329) (160.3177, -47.1632) (159.9137, -47.3957) (159.5105, -47.6306) (159.1083, -47.8677) (158.7069, -48.1071) (158.3064, -48.3486) (157.9068, -48.5923) (157.5081, -48.8381) (157.1103, -49.0861) (156.7134, -49.3361) (156.3173, -49.5882) (155.922, -49.8423) (155.5277, -50.0984) (155.1342, -50.3564) (154.7415, -50.6164) (154.3497, -50.8784) (153.9587, -51.1422) (153.5686, -51.408) (153.1793, -51.6756) (152.7909, -51.9451) (152.4033, -52.2163) (152.0166, -52.4894) (151.6306, -52.7643) (151.2455, -53.041) (150.8613, -53.3194) (150.4778, -53.5996) (150.0952, -53.8815) (149.7134, -54.1651) (149.3325, -54.4504) (148.9523, -54.7374) (148.573, -55.0261) (148.1945, -55.3164) (147.8168, -55.6083) (147.44, -55.9019) (147.0639, -56.1971) (146.6887, -56.4939) (146.3142, -56.7923) (145.9406, -57.0922) (145.5678, -57.3938) (145.1958, -57.6968) (144.8989, -57.9405) (144.6766, -58.124) (144.5285, -58.2466) (144.4545, -58.308) knots 0.13851185 0.13851185 0.13851185 0.13851185 0.13851185 0.13851185 0.14285714 0.15714286 0.17142857 0.18571429 0.2 0.21428571 0.22857143 0.24285714 0.25714286 0.27142857 0.28571429 0.3 0.31428571 0.32857143 0.34285714 0.35714286 0.37142857 0.38571429 0.4 0.41428571 0.42857143 0.44285714 0.45714286 0.47142857 0.48571429 0.5 0.51428571 0.52857143 0.54285714 0.55714286 0.57142857 0.58571429 0.6 0.61428571 0.62857143 0.64285714 0.65714286 0.67142857 0.68571429 0.7 0.71428571 0.72857143 0.74285714 0.75714286 0.77142857 0.78571429 0.8 0.81428571 0.82857143 0.84285714 0.85714286 0.87142857 0.88571429 0.9 0.91428571 0.92857143 0.94285714 0.95714286 0.97142857 0.98571429 1 1 1 1 1 1
  arc A49 (144.4545, -58.308) -> (146.995, -67.7893) centre (452.3696, 19.1166) ccw
  spline S98 degree 5 poles (146.995, -67.7893) (147.0898, -67.8054) (147.2793, -67.8376) (147.5636, -67.8853) (147.9426, -67.9479) (148.4163, -68.0244) (148.8899, -68.0991) (149.3634, -68.1721) (149.8369, -68.2432) (150.3102, -68.3127) (150.7835, -68.3803) (151.2567, -68.4461) (151.7297, -68.5101) (152.2027, -68.5723) (152.6755, -68.6326) (153.1482, -68.6911) (153.6208, -68.7477) (154.0933, -68.8024) (154.5656, -68.8552) (155.0377, -68.9061) (155.5097, -68.9551) (155.9815, -69.0022) (156.4532, -69.0473) (156.9247, -69.0904) (157.396, -69.1315) (157.8671, -69.1707) (158.3381, -69.2078) (158.8088, -69.2429) (159.2793, -69.2759) (159.7496, -69.3069) (160.2196, -69.3357) (160.6895, -69.3625) (161.1591, -69.3871) (161.6284, -69.4095) (162.0974, -69.4298) (162.5662, -69.4478) (163.0347, -69.4636) (163.5029, -69.4772) (163.9708, -69.4884) (164.4384, -69.4973) (164.9057, -69.5039) (165.3726, -69.5082) (165.8392, -69.51) (166.3054, -69.5094) (166.7712, -69.5063) (167.2366, -69.5007) (167.7017, -69.4925) (168.1662, -69.4817) (168.6304, -69.4682) (169.0941, -69.452) (169.5573, -69.4331) (170.02, -69.4114) (170.4823, -69.3869) (170.944, -69.3595) (171.4051, -69.3292) (171.8657, -69.2957) (172.3256, -69.259) (172.7848, -69.2189) (173.2433, -69.1754) (173.7011, -69.1284) (174.1582, -69.078) (174.551, -69.0316) (174.8521, -68.994) (175.0619, -68.9669) (175.1806, -68.9512) (175.2083, -68.9475) knots -1 -1 -1 -1 -1 -1 -0.98571429 -0.97142857 -0.95714286 -0.94285714 -0.92857143 -0.91428571 -0.9 -0.88571429 -0.87142857 -0.85714286 -0.84285714 -0.82857143 -0.81428571 -0.8 -0.78571429 -0.77142857 -0.75714286 -0.74285714 -0.72857143 -0.71428571 -0.7 -0.68571429 -0.67142857 -0.65714286 -0.64285714 -0.62857143 -0.61428571 -0.6 -0.58571429 -0.57142857 -0.55714286 -0.54285714 -0.52857143 -0.51428571 -0.5 -0.48571429 -0.47142857 -0.45714286 -0.44285714 -0.42857143 -0.41428571 -0.4 -0.38571429 -0.37142857 -0.35714286 -0.34285714 -0.32857143 -0.31428571 -0.3 -0.28571429 -0.27142857 -0.25714286 -0.24285714 -0.22857143 -0.21428571 -0.2 -0.18571429 -0.17142857 -0.15714286 -0.14285714 -0.13851185 -0.13851185 -0.13851185 -0.13851185 -0.13851185 -0.13851185
  spline S99 degree 3 poles (176.928, -70.0323) (176.8643, -69.8356) (176.7629, -69.6532) (176.4958, -69.3377) (176.3327, -69.2075) (176.0054, -69.0376) (175.851, -68.9853) (175.5318, -68.9295) (175.3689, -68.9261) (175.2083, -68.9475) knots 0 0 0 0 0.062015 0.062015 0.12403 0.12403 0.172638 0.172638 0.221247 0.221247 0.221247 0.221247
  arc A50 (176.928, -70.0323) -> (179.5767, -77.8351) centre (452.3696, 19.1166) ccw
  spline S100 degree 3 poles (178.8727, -79.7426) (179.0519, -79.6395) (179.2092, -79.5024) (179.4624, -79.1755) (179.5559, -78.989) (179.6541, -78.6335) (179.6731, -78.4717) (179.6615, -78.1478) (179.6309, -77.9877) (179.5767, -77.8351) knots 0 0 0 0 0.062015 0.062015 0.12403 0.12403 0.172638 0.172638 0.221247 0.221247 0.221247 0.221247
  spline S101 degree 5 poles (178.8727, -79.7426) (178.8485, -79.7565) (178.7448, -79.8163) (178.5618, -79.9225) (178.3001, -80.076) (177.9602, -80.2783) (177.5668, -80.5166) (177.1751, -80.758) (176.7848, -81.0025) (176.3961, -81.2503) (176.0089, -81.5011) (175.6231, -81.755) (175.2388, -82.0116) (174.8558, -82.271) (174.4742, -82.5329) (174.0939, -82.7974) (173.7149, -83.0644) (173.3372, -83.3339) (172.9607, -83.6057) (172.5855, -83.8799) (172.2116, -84.1565) (171.839, -84.4354) (171.4675, -84.7166) (171.0973, -84.9999) (170.7282, -85.2854) (170.3604, -85.573) (169.9937, -85.8626) (169.6282, -86.1544) (169.2638, -86.4481) (168.9006, -86.7439) (168.5385, -87.0417) (168.1776, -87.3413) (167.8178, -87.643) (167.4591, -87.9465) (167.1016, -88.2519) (166.7451, -88.5591) (166.3897, -88.8681) (166.0355, -89.179) (165.6823, -89.4916) (165.3302, -89.806) (164.9792, -90.1221) (164.6293, -90.44) (164.2804, -90.7595) (163.9326, -91.0808) (163.5858, -91.4037) (163.2402, -91.7283) (162.8955, -92.0545) (162.5519, -92.3823) (162.2094, -92.7117) (161.8679, -93.0427) (161.5274, -93.3753) (161.188, -93.7095) (160.8496, -94.0452) (160.5122, -94.3824) (160.1759, -94.7212) (159.8405, -95.0614) (159.5062, -95.4032) (159.173, -95.7464) (158.8407, -96.0911) (158.5094, -96.4373) (158.1792, -96.7849) (157.8499, -97.1339) (157.5873, -97.4143) (157.3908, -97.6252) (157.26, -97.7661) (157.1947, -97.8366) knots 0.13851185 0.13851185 0.13851185 0.13851185 0.13851185 0.13851185 0.14285714 0.15714286 0.17142857 0.18571429 0.2 0.21428571 0.22857143 0.24285714 0.25714286 0.27142857 0.28571429 0.3 0.31428571 0.32857143 0.34285714 0.35714286 0.37142857 0.38571429 0.4 0.41428571 0.42857143 0.44285714 0.45714286 0.47142857 0.48571429 0.5 0.51428571 0.52857143 0.54285714 0.55714286 0.57142857 0.58571429 0.6 0.61428571 0.62857143 0.64285714 0.65714286 0.67142857 0.68571429 0.7 0.71428571 0.72857143 0.74285714 0.75714286 0.77142857 0.78571429 0.8 0.81428571 0.82857143 0.84285714 0.85714286 0.87142857 0.88571429 0.9 0.91428571 0.92857143 0.94285714 0.95714286 0.97142857 0.98571429 1 1 1 1 1 1
  arc A51 (157.1947, -97.8366) -> (160.951, -106.9052) centre (452.3696, 19.1166) ccw
  spline S102 degree 5 poles (160.951, -106.9052) (161.0471, -106.9088) (161.2392, -106.916) (161.5273, -106.9262) (161.9112, -106.9387) (162.3908, -106.9527) (162.8701, -106.965) (163.3491, -106.9755) (163.8278, -106.9843) (164.3062, -106.9913) (164.7843, -106.9966) (165.262, -107.0001) (165.7393, -107.0018) (166.2164, -107.0017) (166.693, -106.9998) (167.1693, -106.9961) (167.6452, -106.9905) (168.1208, -106.9831) (168.5959, -106.9738) (169.0707, -106.9627) (169.545, -106.9496) (170.019, -106.9347) (170.4925, -106.9178) (170.9656, -106.8991) (171.4383, -106.8783) (171.9105, -106.8557) (172.3822, -106.831) (172.8535, -106.8043) (173.3243, -106.7757) (173.7946, -106.745) (174.2644, -106.7122) (174.7337, -106.6774) (175.2024, -106.6405) (175.6707, -106.6015) (176.1384, -106.5603) (176.6055, -106.517) (177.0721, -106.4716) (177.538, -106.4239) (178.0034, -106.374) (178.4681, -106.3218) (178.9323, -106.2673) (179.3957, -106.2106) (179.8586, -106.1515) (180.3207, -106.09) (180.7821, -106.0262) (181.2429, -105.9599) (181.7028, -105.891) (182.162, -105.8197) (182.6205, -105.7457) (183.0781, -105.6691) (183.5348, -105.5899) (183.9908, -105.508) (184.4459, -105.4234) (184.9001, -105.336) (185.3533, -105.2457) (185.8056, -105.1524) (186.2567, -105.056) (186.7068, -104.9563) (187.1557, -104.8533) (187.6034, -104.747) (188.05, -104.6373) (188.4334, -104.5401) (188.7271, -104.4635) (188.9315, -104.4092) (189.0471, -104.3781) (189.0741, -104.3709) knots -1 -1 -1 -1 -1 -1 -0.98571429 -0.97142857 -0.95714286 -0.94285714 -0.92857143 -0.91428571 -0.9 -0.88571429 -0.87142857 -0.85714286 -0.84285714 -0.82857143 -0.81428571 -0.8 -0.78571429 -0.77142857 -0.75714286 -0.74285714 -0.72857143 -0.71428571 -0.7 -0.68571429 -0.67142857 -0.65714286 -0.64285714 -0.62857143 -0.61428571 -0.6 -0.58571429 -0.57142857 -0.55714286 -0.54285714 -0.52857143 -0.51428571 -0.5 -0.48571429 -0.47142857 -0.45714286 -0.44285714 -0.42857143 -0.41428571 -0.4 -0.38571429 -0.37142857 -0.35714286 -0.34285714 -0.32857143 -0.31428571 -0.3 -0.28571429 -0.27142857 -0.25714286 -0.24285714 -0.22857143 -0.21428571 -0.2 -0.18571429 -0.17142857 -0.15714286 -0.14285714 -0.13851185 -0.13851185 -0.13851185 -0.13851185 -0.13851185 -0.13851185
  spline S103 degree 3 poles (190.9207, -105.2219) (190.8319, -105.0352) (190.7075, -104.8677) (190.4015, -104.5897) (190.2228, -104.4819) (189.8762, -104.3561) (189.7163, -104.3245) (189.3925, -104.3108) (189.2305, -104.3287) (189.0741, -104.3709) knots 0 0 0 0 0.062015 0.062015 0.12403 0.12403 0.172638 0.172638 0.221247 0.221247 0.221247 0.221247
  arc A52 (190.9207, -105.2219) -> (194.5652, -112.6123) centre (452.3696, 19.1166) ccw
  spline S104 degree 3 poles (194.1162, -114.5953) (194.2804, -114.4697) (194.4185, -114.3132) (194.6268, -113.9562) (194.6952, -113.759) (194.7462, -113.3938) (194.7439, -113.2308) (194.6901, -112.9113) (194.6389, -112.7565) (194.5652, -112.6123) knots 0 0 0 0 0.062015 0.062015 0.12403 0.12403 0.172638 0.172638 0.221247 0.221247 0.221247 0.221247